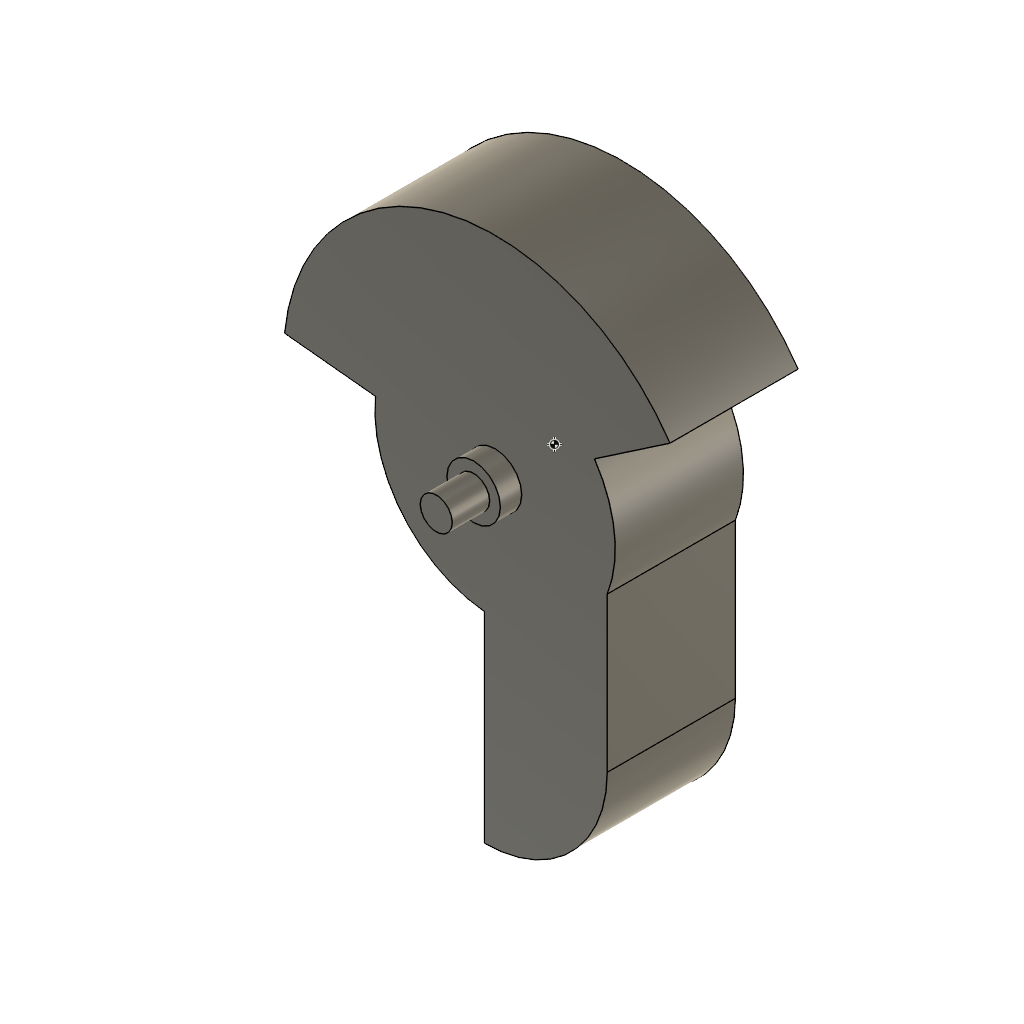
weapon (Autodesk Fusion 360 design; units mm, degrees)
Autodesk Fusion 360 part; units mm, degrees
sketch "Sketch1" plane through (0, 0, 0) normal (0, 1, 0) x (1, 0, 0)
  circle A0 centre (0, 0) radius 22.5
  circle A1 centre (0, 0) radius 39.6
  circle A2 centre (0, 0) radius 60
  arc A3 (-9.2591, -13.6269) -> (-9.0527, -14.0335) centre (-8.81, -13.6546) ccw
  arc A4 (-0.7038, -14.8834) -> (-1.1218, -15.0774) centre (-0.726, -15.3829) ccw
  arc A5 (-9.1509, -12.0328) -> (-9.3379, -11.611) centre (-9.6499, -12.0016) ccw
  arc A6 (8.9275, 13.8422) -> (8.7141, 14.2462) centre (8.478, 13.8631) ccw
  arc A7 (-2.5253, -16.508) -> (-2.1019, -16.3377) centre (-2.4583, -16.063) ccw
  line L0 (1.709, 16.3855) -> (0.765, 15.098)
  arc A8 (-9.0527, -14.0335) -> (-2.5253, -16.508) centre (0, 0) ccw
  arc A9 (8.7141, 14.2462) -> (2.1296, 16.5637) centre (0, 0) ccw
  arc A10 (2.1296, 16.5637) -> (1.709, 16.3855) centre (2.0705, 16.1176) ccw
  line L1 (-2.1019, -16.3377) -> (-1.1218, -15.0774)
  line L2 (8.8652, 12.2481) -> (8.9275, 13.8422)
  line L3 (-9.1509, -12.0328) -> (-9.2591, -13.6269)
  arc A11 (0.3491, 14.8959) -> (0.765, 15.098) centre (0.3633, 15.3957) ccw
  circle A12 centre (0, 0) radius 13.9
  arc A13 (-0.7038, -14.8834) -> (9.0593, 11.8296) centre (0, 0) ccw
  arc A14 (8.8652, 12.2481) -> (9.0593, 11.8296) centre (9.3647, 12.2255) ccw
  arc A15 (0.3491, 14.8959) -> (-9.3379, -11.611) centre (0, 0) ccw
  line L4 (-39.3975, -3.9999) -> (0, 0)
  line L5 (0, 0) -> (32.7513, -22.2601)
  line L6 (0, 0) -> (0, 60)
  line L7 (-2, 36.9667) -> (21, 36.9667)
  line L8 (-2, 36.9667) -> (-2, 22.4109)
  line L9 (21, 36.9667) -> (21, 8.0777)
  line L10 (-2, 36.9667) -> (-2, 59.9667)
  arc A16 (21, 36.9667) -> (-2, 59.9667) centre (-2, 36.9667) ccw
  circle A17 centre (0, 0) radius 5.5
  circle A18 centre (0, 0) radius 15.4
  point P0 (-2, 36.9667)
  dimension "d1" = 45
  dimension "d2" = 79.2
  dimension "d3" = 120
  dimension "d4" = 14.9
  dimension "d5" = 14.9
  dimension "d6" = 16.7
  dimension "d7" = 16.7
  dimension "d8" = 0.5
  dimension "d9" = 0.45
  dimension "d10" = 0.45
  dimension "d11" = 0.5
  dimension "d12" = 1.5942
  dimension "d13" = 1.5965
  dimension "d14" = 7.6534
  dimension "d15" = 8.5869
  dimension "d16" = 1.5965
  dimension "d17" = 0.5
  dimension "d18" = 0.45
  dimension "d20" = 1.5942
  dimension "d21" = 0.5
  dimension "d22" = 0.45
  dimension "d23" = 8.5869
  dimension "d24" = 7.6534
  dimension "d25" = 140
  dimension "d29" = 11
  dimension "d46" = 23
  dimension "d48" = 2
  dimension "d49" = 30.8
  constraint coincident A0.centre A1.centre
  constraint concentric A1 A2
  constraint coincident A1 L4.start
  constraint perpendicular A1 L4
  constraint coincident A1 L5.end
  constraint coincident A2 L6.end
  constraint perpendicular L6 L7
  constraint parallel L8 L9
  constraint coincident A0 L9.end
  constraint parallel L6 L8
  constraint coincident A2 L10.end
  constraint perpendicular L7 L10
  constraint tangent L9 A16
  constraint perpendicular L10 A16
  constraint coincident A0 L8.end
  constraint coincident P0 L7.start
  constraint vertical L10
  constraint concentric A1 A17
  measures "d1" diameter of A0
  measures "d2" diameter of A1
  measures "d3" diameter of A2
  measures "d4" radius of A13
  measures "d5" radius of A15
  measures "d6" radius of A8
  measures "d7" radius of A9
  measures "d8" radius of A5
  measures "d9" radius of A3
  measures "d10" radius of A7
  measures "d11" radius of A4
  measures "d12" vertical distance of A5.start A3.start
  measures "d13" distance of A7.end A4.end
  measures "d14" distance of A3.start A7.end
  measures "d15" distance of A5.start A4.end
  measures "d16" distance of L0.end L0.start
  measures "d17" radius of A11
  measures "d18" radius of A10
  measures "d20" vertical distance of L2.start A6.start
  measures "d21" radius of A14
  measures "d22" radius of A6
  measures "d23" distance of L0.end L2.start
  measures "d24" distance of L0.start A6.start
  measures "d25" angle of L4 L5
  measures "d29" diameter of A17
  measures "d46" distance of L8 L9
  measures "d48" distance of L6 L8
  measures "d49" diameter of A18
extrude "Extrude1" add sketch "Sketch1" along normal blind 13 contours A0 A6 L0 A9 A10 L2 L5 L6 A18 | A0 A1 L6 L7 L9 | A0 A1 L4 L5 | A0 A3 A7 A8 L1 L3 L4 L5 A18 | A0 L4 L6 A18 | A0 L6 L7 L8 | A1 L7 L9 | A1 L6 L7 L10 | A1 L6 L7 | A1 L6 L7 A16 | A1 L6 L10 A16
extrude "Extrude2" add sketch "Sketch1" against normal blind 3 contours A0 A6 L0 A9 A10 L2 L5 L6 A18 | A0 A1 L6 L7 L9 | A0 A1 L4 L5 | A0 A3 A7 A8 L1 L3 L4 L5 A18 | A0 L4 L6 A18 | A0 L6 L7 L8 | A1 L7 L9 | A4 L1 A13 L5 A18 | L2 A13 A14 L5 A18 | L0 A11 A15 L6 A18 | A15 L4 L6 A18 | A1 L6 L7 L10 | A1 L6 L7 | A1 L6 L7 A16 | A5 L3 A15 L4 A18 | L0 L2 A11 A12 A13 A14 A15 L5 L6 A18 | A4 A5 L1 L3 A12 A13 A15 L4 L5 A18 | A3 A7 A8 L1 L3 A18 | A12 A15 L4 L6 | A6 L0 A9 A10 L2 A18 | A1 L6 L10 A16 | A12 L5 L6 A17 | A12 L4 L5 A17 | A12 L4 L6 A17
sketch "Sketch2" plane through (0, -3, 0) normal (0, -1, 0) x (1, 0, 0)
  line L0 (21, -36.9667) -> (21, -8.0777)
  arc A0 (21, -8.0777) -> (18.6087, 12.6478) centre (0, 0) ccw
  line L1 (-2, -22.4109) -> (-2, -59.9667)
  arc A1 (-2, -59.9667) -> (21, -36.9667) centre (-2, -36.9667) ccw
  circle A2 centre (0, 0) radius 2.5
  circle A3 centre (0, 0) radius 4.5
  circle A4 centre (0, 0) radius 5.5
  line L2 (18.6087, 12.6478) -> (32.7513, 22.2601)
  arc A5 (32.7513, 22.2601) -> (-39.3975, 3.9999) centre (0, 0) ccw
  line L3 (-39.3975, 3.9999) -> (-22.3849, 2.2727)
  arc A6 (-22.3849, 2.2727) -> (-2, -22.4109) centre (0, 0) ccw
  dimension "d32" = 5
  dimension "d41" = 9
  constraint concentric A2 A3
  measures "d32" diameter of A2
  measures "d41" diameter of A3
extrude "Extrude3" add sketch "Sketch2" along normal blind 8 contours L0 A0 L1 A1 L2 A5 L3 A6 | A3 | A4
sketch "Sketch4" plane through (0, -11, 0) normal (0, -1, 0) x (1, 0, 0)
  arc A0 (-2, -59.9667) -> (21, -36.9667) centre (-2, -36.9667) ccw
  line L0 (21, -36.9667) -> (21, -8.0777)
  arc A1 (21, -8.0777) -> (18.6087, 12.6478) centre (0, 0) ccw
  line L1 (-2, -22.4109) -> (-2, -59.9667)
  circle A2 centre (0, 0) radius 2.5
  circle A3 centre (0, 0) radius 5
  circle A4 centre (0, 0) radius 2.5
  line L2 (18.6087, 12.6478) -> (32.7513, 22.2601)
  arc A5 (32.7513, 22.2601) -> (-39.3975, 3.9999) centre (0, 0) ccw
  line L3 (-39.3975, 3.9999) -> (-22.3849, 2.2727)
  arc A6 (-22.3849, 2.2727) -> (-2, -22.4109) centre (0, 0) ccw
  dimension "d42" = 10
  constraint coincident A1.centre A2.centre
  measures "d42" diameter of A3
extrude "Extrude4" add sketch "Sketch4" along normal blind 2 contours A3
sketch "Sketch5" plane through (0, -13, 0) normal (0, -1, 0) x (1, 0, 0)
  circle A0 centre (0, 0) radius 2
  circle A1 centre (0, 0) radius 2.5
  circle A2 centre (0, 0) radius 5
  dimension "d38" = 4
  measures "d38" diameter of A0
extrude "Extrude5" add sketch "Sketch5" along normal blind 2 contours A0 | A1 | A2
sketch "Sketch6" plane through (0, -15, 0) normal (0, -1, 0) x (1, 0, 0)
  circle A0 centre (0, 0) radius 5
  circle A1 centre (0, 0) radius 3
  dimension "d43" = 6
  constraint coincident A0.centre A1.centre
  measures "d43" diameter of A1
extrude "Extrude6" add sketch "Sketch6" along normal blind 7 contours A1
equation "d49 = 15.4 * 2 mm"
